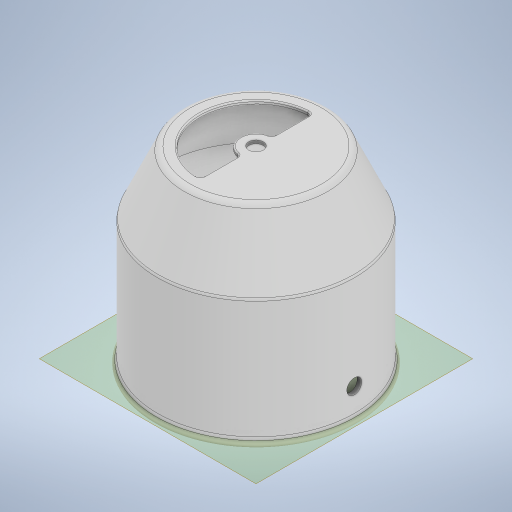
# Autodesk Inventor part: ikea watering can - pt base
Saved by Autodesk Inventor 2024 (Build 280153000, 153)
## iProperties
Created: 2025-01-25
Part Number: ikea watering can - pt base
Material: Generic
Document SubType Name: Modeling
Designer: haque
Density: 1 g/cm^3
Appearance: Default
Author: haque
Autodesk Inventor part; units mm, degrees
sketch "Sketch1" plane through (0, 0, 0) normal (0, 1, 0) x (-1, 0, 0)
  circle A0 centre (0, 0) radius 80
  dimension "d0" = 160
  constraints: 1 centre point, 1 coincident
  measures "d0" diameter of A0
extrude "Extrusion1" add sketch "Sketch1" along normal blind 5
fillet "Fillet1" radius 2.5 2 edges at (80, 5, 0) (80, 0, 0)
sketch "Sketch2" plane through (0, 5, 0) normal (0, 1, 0) x (1, 0, 0)
  circle A0 centre (0, 0) radius 77.5 projected
  circle A1 centre (0, 0) radius 74
  dimension "d4" = 148
  constraints: 1 centre point, 1 coincident
  measures "d4" diameter of A1
extrude "Extrusion2" add sketch "Sketch2" along normal blind 95
ref_plane "Work Plane1" through (0, 150, 0) normal (0, 1, 0) x (1, 0, 0)
sketch "Sketch3" plane through (0, 150, 0) normal (0, 1, 0) x (1, 0, 0)
  circle A0 centre (0, 0) radius 55
  circle A1 centre (0, 0) radius 51.5
  point P0 (51.5, 0)
  point P1 (55, 0)
  point P2 (0, 51.5)
  point P3 (0, 55)
  dimension "d8" = 110
  dimension "d9" = 103
  constraints: 4 point on circle, 2 centre point, 2 coincident
  measures "d8" diameter of A0
  measures "d9" diameter of A1
extrude "Extrusion3" add sketch "Sketch3" against normal blind 3.5 contours A0 | A1
sketch "Sketch5" plane through (0, 100, 0) normal (0, 1, 0) x (1, 0, 0)
  circle A0 centre (0, 0) radius 74 projected
  circle A1 centre (0, 0) radius 77.5 projected
  point P0 (74, 0)
  point P1 (77.5, 0)
  constraints: 2 horizontal alignment, 2 other
sketch "Sketch6" plane through (0, 0, 0) normal (0, 0, 1) x (1, 0, 0)
  line L0 (-74, 100) -> (74, 100) projected
  line L1 (77.5, 100) -> (-77.5, 100) projected
  line L2 (74, 100) -> (77.5, 100)
  line L3 (55, 150) -> (-55, 150) projected
  line L4 (55, 150) -> (51.5, 150)
  line L5 (51.5, 150) -> (74, 100)
  line L6 (55, 150) -> (77.5, 100)
  line L7 (0, -30) -> (0, 180) projected
  point P0 (0, 0)
  dimension "d12" = 3.5
  constraints: 8 end point, 1 horizontal, 1 point on line
  measures "d12" distance of L3.start L4.end
revolve "Revolution1" add sketch "Sketch6" angle 360 about axis through (0, -10, 0) along (0, 1, 0) contours L5 L3 L6 L1
sketch "Sketch7" plane through (0, 150, 0) normal (0, 1, 0) x (1, 0, 0)
  arc A0 (0, -12.5) -> (0, 12.5) centre (0, 0) ccw
  arc A1 (0, -44) -> (0, 44) centre (0, 0) ccw
  line L0 (0, 44) -> (0, -44)
  dimension "d14" = 25
  dimension "d15" = 88
  dimension "d16" = 88
  constraints: 4 point on circle, 2 centre point, 2 coincident, 2 end point, 2 point on line, 1 vertical
  measures "d14" diameter of A0
  measures "d15" diameter of A1
  measures "d16" distance of L0.start L0.end
extrude "Extrusion4" cut sketch "Sketch7" against normal blind 3.5 contours A0 L0 A1
sketch "Sketch8" plane through (0, 150, 0) normal (0, 1, 0) x (1, 0, 0)
  circle A0 centre (0, 0) radius 5.75
  dimension "d19" = 11.5
  constraints: 1 centre point, 1 coincident
  measures "d19" diameter of A0
ref_plane "Work Plane2" through (77.5, 0, 0) normal (1, 0, 0) x (0, 1, 0)
sketch "Sketch9" plane through (77.5, 0, 0) normal (1, 0, 0) x (0, 1, 0)
  line L0 (100, 74) -> (100, -74) projected
  line L1 (100, 0) -> (0, 0)
  line L2 (0, -77.5) -> (0, 77.5) projected
  line L3 (100, 0) -> (50, 0)
  line L4 (50, 0) -> (25, 0)
  circle A0 centre (25, 0) radius 5
  dimension "d21" = 25
  dimension "d22" = 10
  constraints: 6 end point, 3 coincident, 2 midpoint, 1 centre point, 1 perpendicular, 1 point on line
  measures "d21" distance of L4.start L4.end
  measures "d22" diameter of A0
fillet "Fillet2" radius 3 4 edges at (0, 148.25, -44) (0, 148.25, 12.5) (0, 148.25, 44) (0, 148.25, -12.5)
fillet "Fillet3" radius 1 16 edges at (0.9578, 150, -43.0877) (44, 150, 0) (0.9578, 150, 43.0877) (0, 150, 28.0485) (0.6825, 150, 13.3019) (12.5, 150, 0) (0.6825, 150, -13.3019) (0, 150, -28.0485) (0.6825, 146.5, -13.3019) (12.5, 146.5, 0) (0.6825, 146.5, 13.3019) (0, 146.5, 28.0485) (0.9578, 146.5, 43.0877) (44, 146.5, 0) (0.9578, 146.5, -43.0877) (0, 146.5, -28.0485)
sketch "Sketch11" plane through (0, 0, 0) normal (0, 0, 1) x (1, 0, 0)
  line L0 (0, 149) -> (0, 147.5) projected
  line L1 (0, 149) -> (0, 184)
  line L2 (-74, 100) -> (74, 100) projected
  line L3 (77.5, 5) -> (77.5, 100) projected
  line L4 (77.5, 25) -> (77.5, -10)
  line L5 (77.5, -10) -> (77.5, 25)
  line L6 (77.5, 25) -> (117.5, 25)
  line L7 (117.5, 25) -> (117.5, 184)
  line L8 (117.5, 184) -> (0, 184)
  line L9 (0, 149) -> (0, 166.5)
  line L10 (0, 149) -> (0, 159)
  line L11 (77.5, 25) -> (91.25, 25)
  line L12 (117.5, 184) -> (91.25, 184)
  line L13 (117.5, 184) -> (117.5, 157.75)
  line L14 (0, 149) -> (0, 157.75)
  line L15 (117.5, 25) -> (117.5, 51.25)
  line L16 (0, 184) -> (26.25, 184)
  arc A0 (26.25, 184) -> (0, 157.75) centre (26.25, 157.75) ccw
  arc A1 (117.5, 157.75) -> (91.25, 184) centre (91.25, 157.75) ccw
  arc A2 (91.25, 25) -> (117.5, 51.25) centre (91.25, 51.25) ccw
  line L17 (26.25, 184) -> (91.25, 184)
  line L18 (117.5, 157.75) -> (117.5, 51.25)
  line L19 (91.25, 25) -> (77.5, 25)
  line L20 (77.5, 25) -> (75.75, 25)
  line L21 (74, 100) -> (74, 5) projected
  line L22 (55, 150) -> (-55, 150) projected
  line L23 (0, 150) -> (0, 148.25)
  line L24 (0, 149) -> (0, 147.5) projected
  point P0 (0, 0)
  point P1 (0, 157.75)
  dimension "d25" = 35
  dimension "d26" = 35
  dimension "d27" = 40
  dimension "d28" = 10
  dimension "d29" = 13.75
  dimension "d30" = 26.25
  dimension "d31" = 26.25
  dimension "d32" = 75
  dimension "d33" = 8.75
  dimension "d34" = 26.25
  dimension "d35" = 26.25
  dimension "d36" = 26.25
  dimension "d37" = 26.25
  dimension "d38" = 26.25
  dimension "d77" = 1.75
  dimension "d78" = 15.5
  dimension "d79" = 1.75
  dimension "d80" = 9.5
  constraints: 38 end point, 8 point on line, 6 point on circle, 5 collinear, 5 midpoint, 5 perpendicular, 4 coincident, 3 centre point, 1 tangent
  measures "d25" distance of L0.start L1.end
  measures "d26" distance of L4.start L4.end
  measures "d27" distance of L4.start L6.end
  measures "d28" distance of L0.start L10.end
  measures "d29" distance of L4.start L11.end
  measures "d30" distance of L7.end L12.end
  measures "d31" distance of L7.end L13.end
  measures "d32" distance between parallel lines of L2 L6
  measures "d33" distance of L0.start L14.end
  measures "d34" distance of point (0, 157.75) L1.end
  measures "d35" distance of L15.end L6.end
  measures "d36" distance of L8.end L16.end
  measures "d37" distance from line of L7 point (91.25, 157.75)
  measures "d38" distance from line of L7 point (91.25, 51.25)
  measures "d77" distance of L4.start L20.end
  measures "d78" distance of L11.end L20.end
  measures "d79" distance of L23.start L23.end
  measures "d80" distance of point (0, 157.75) point (0, 148.25)
sketch "Sketch12" plane through (0, 150, 0) normal (0, 1, 0) x (1, 0, 0)
  circle A0 centre (0, 0) radius 5
  dimension "d39" = 10
  constraints: 1 centre point, 1 coincident
  measures "d39" diameter of A0
extrude "Extrusion5" add sketch "Sketch12" along normal blind 0.5
sweep "Sweep1" cut profiles "Sketch8" path "Sketch11" path curves L24 L14 A0 L17 A1 L18 A2 L11 L20
ref_plane "Work Plane3" through (-77.5, 0, 0) normal (1, 0, 0) x (0, 1, 0)
sketch "Sketch13" plane through (-77.5, 0, 0) normal (1, 0, 0) x (0, 1, 0)
  line L0 (100, 74) -> (100, -74) projected
  line L1 (100, 0) -> (25, 0)
  line L2 (25, 0) -> (5, 0)
  line L3 (5, -74) -> (5, 74) projected
  circle A0 centre (25, 0) radius 5.75
  point P0 (0, 0)
  dimension "d45" = 75
  dimension "d46" = 11.5
  constraints: 4 end point, 2 midpoint, 1 centre point, 1 coincident, 1 horizontal
  measures "d45" distance of L1.start L1.end
  measures "d46" diameter of A0
ref_plane "Work Plane4" through (-252.5, 0, 0) normal (1, 0, 0) x (0, 1, 0)
sketch "Sketch17" plane through (-77.5, 0, 0) normal (1, 0, 0) x (0, 1, 0)
  line L0 (19.25, 0) -> (30.75, 0) projected
  circle A0 centre (25, 0) radius 5.85
  point P0 (0, 0)
  point P1 (20, 0)
  point P2 (30, 0)
  dimension "d76" = 11.7
  constraints: 1 centre point, 1 midpoint
  measures "d76" diameter of A0
extrude "Extrusion7" cut sketch "Sketch17" along normal blind 5
fillet "Fillet4" radius 2 2 edges at (0, 5, -77.5001) (0, 5, 77.5001)
fillet "Fillet5" radius 5 2 edges at (-77.5, 100, 0) (-55, 150, 0)
ref_plane "Work Plane5" through (0, 5, 0) normal (0, -1, 0) x (1, 0, 0)
body "Solid1"
